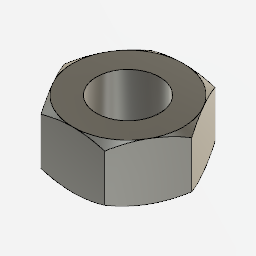
HEX_Nut (Autodesk Fusion 360 design; units mm, degrees)
Autodesk Fusion 360 part; units mm, degrees
sketch "Sketch1" plane through (0, 0, 0) normal (0, 0, 1) x (1, 0, 0)
  circle A0 centre (0, 0) radius 3.175
  line L0 (-6.4231, 0) -> (-3.2116, -5.5626)
  line L1 (-3.2116, -5.5626) -> (3.2116, -5.5626)
  line L2 (3.2116, -5.5626) -> (6.4231, 0)
  line L3 (6.4231, 0) -> (3.2116, 5.5626)
  line L4 (3.2116, 5.5626) -> (-3.2116, 5.5626)
  line L5 (-3.2116, 5.5626) -> (-6.4231, 0)
  dimension "diameter" = 6.35
  dimension "hexwidth" = 11.1252
  measures "diameter" diameter of A0
  measures "hexwidth" distance of L1 L4
extrude "Extrude1" add sketch "Sketch1" along normal blind 5.7404
sketch "Sketch2" plane through (0, 0, 5.7404) normal (0, 0, 1) x (-1, 0, 0)
  circle A0 centre (0, 0) radius 3.175 construction
  line L0 (3.2116, -5.5626) -> (6.4231, 0) construction
  line L1 (6.4231, 0) -> (3.2116, 5.5626) construction
  line L2 (3.2116, 5.5626) -> (-3.2116, 5.5626) construction
  line L3 (-3.2116, 5.5626) -> (-6.4231, 0) construction
  line L4 (-6.4231, 0) -> (-3.2116, -5.5626) construction
  line L5 (-3.2116, -5.5626) -> (3.2116, -5.5626) construction
  circle A1 centre (0, 0) radius 5.5626
  circle A2 centre (0, 0) radius 30.9626
  dimension "hexcutoffset2" = 25.4
  measures "hexcutoffset2" distance of A1 A2
extrude "Extrude2" cut sketch "Sketch2" against normal blind 0.7366 draft -60
sketch "Sketch3" plane through (0, 0, 0) normal (0, 0, -1) x (1, 0, 0)
  circle A0 centre (0, 0) radius 3.175 construction
  line L0 (-6.4231, 0) -> (-3.2116, -5.5626) construction
  line L1 (-3.2116, -5.5626) -> (3.2116, -5.5626) construction
  line L2 (3.2116, -5.5626) -> (6.4231, 0) construction
  line L3 (6.4231, 0) -> (3.2116, 5.5626) construction
  line L4 (3.2116, 5.5626) -> (-3.2116, 5.5626) construction
  line L5 (-3.2116, 5.5626) -> (-6.4231, 0) construction
  circle A1 centre (0, 0) radius 5.5626
  circle A2 centre (0, 0) radius 30.9626
  dimension "hexcutoffset1" = 25.4
  measures "hexcutoffset1" distance of A1 A2
extrude "Extrude3" cut sketch "Sketch3" against normal blind 1.0414 draft -60
equation "thickness = 0.226 in"
equation "hexcut1 = -0.029 in"
equation "hexcut2 = -0.041 in"
